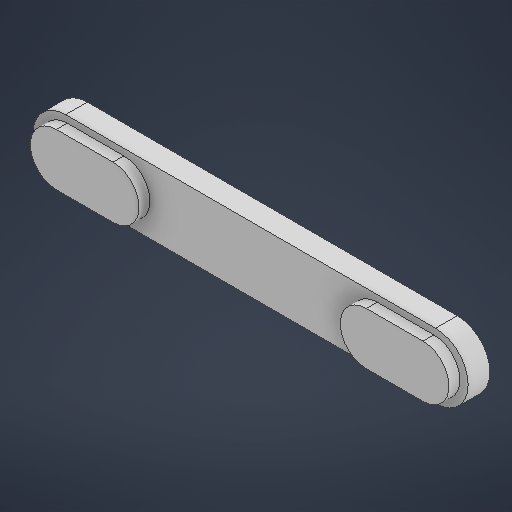
# Autodesk Inventor part: 音量接口
Saved by Autodesk Inventor 2025 (Build 290162000, 162)
## iProperties
Created: 2025-11-17
Part Number: 音量接口
Material: 常规
Document SubType Name: Modeling
Designer: XH
Density: 1 g/cm^3
Appearance: 默认
Author: XH
Autodesk Inventor part; units mm, degrees
ref_plane "YZ Plane" through (0, 0, 0) normal (1, 0, 0) x (0, 1, 0)
ref_plane "XZ Plane" through (0, 0, 0) normal (0, 1, 0) x (-1, 0, 0)
ref_plane "XY Plane" through (0, 0, 0) normal (0, 0, 1) x (1, 0, 0)
sketch "草图1" plane through (0, 0, 0) normal (0, 0, 1) x (1, 0, 0)
  line L0 (-8.5, 0) -> (8.5, 0) construction
  line L1 (-8.5, -1.5) -> (8.5, -1.5)
  line L2 (8.5, 1.5) -> (-8.5, 1.5)
  arc A0 (-8.5, 1.5) -> (-8.5, -1.5) centre (-8.5, 0) ccw
  arc A1 (8.5, -1.5) -> (8.5, 1.5) centre (8.5, 0) ccw
  line L3 (5.8209, 0) -> (8.4219, 0) construction
  line L4 (5.8209, -1.1995) -> (8.4219, -1.1995)
  line L5 (8.4219, 1.1995) -> (5.8209, 1.1995)
  arc A2 (5.8209, 1.1995) -> (5.8209, -1.1995) centre (5.8209, 0) ccw
  arc A3 (8.4219, -1.1995) -> (8.4219, 1.1995) centre (8.4219, 0) ccw
  line L6 (0, 2.5577) -> (0, -3.2218)
  line L7 (-5.8209, 0) -> (-8.4219, 0) construction
  line L8 (-5.8209, -1.1995) -> (-8.4219, -1.1995)
  line L9 (-8.4219, 1.1995) -> (-5.8209, 1.1995)
  arc A4 (-5.8209, -1.1995) -> (-5.8209, 1.1995) centre (-5.8209, 0) ccw
  arc A5 (-8.4219, 1.1995) -> (-8.4219, -1.1995) centre (-8.4219, 0) ccw
  point P0 (0, 0)
  point P1 (-10, 0)
  point P2 (10, 0)
  point P3 (7.1214, 0)
  point P4 (4.6214, 0)
  point P5 (9.6214, 0)
  point P6 (-7.1214, 0)
  point P7 (-4.6214, 0)
  point P8 (-9.6214, 0)
  dimension "d0" = 20
  dimension "d1" = 3
  dimension "d2" = 5
  constraints: 26 end point, 16 point on circle, 9 symmetric about line, 8 tangent, 6 centre point, 2 midpoint, 2 parallel, 2 point on line, 1 horizontal, 1 vertical, 2 other
  measures "d0" distance of point (-10, 0) point (10, 0)
  measures "d1" distance between parallel lines of L1 L2
  measures "d2" distance of point (4.621, 0) point (9.621, 0)
extrude "拉伸1" add sketch "草图1" along normal blind 1
extrude "拉伸2" add sketch "草图1" along normal blind 1.5 contours A2 L5 A3 L4 | L8 A5 L9 A4
